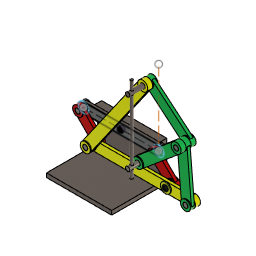
mechanism (Autodesk Fusion 360 design; units mm, degrees)
Autodesk Fusion 360 part; units mm, degrees
sketch "holder" plane through (0, 0, 0) normal (0, 1, 0) x (1, 0, 0) in component "holder"
  line L0 (-37.5, -5) -> (37.5, -5)
  arc A0 (37.5, -5) -> (37.5, 5) centre (37.5, 0) ccw
  line L1 (37.5, 5) -> (-37.5, 5)
  arc A1 (-37.5, 5) -> (-37.5, -5) centre (-37.5, 0) ccw
  line L2 (-37.5, 0) -> (37.5, 0) construction
  circle A2 centre (-37.5, 0) radius 5
  circle A3 centre (-37.5, 0) radius 2.5
  circle A4 centre (37.5, 0) radius 5
  circle A5 centre (37.5, 0) radius 2.5
  line L3 (37.5, 0) -> (37.5, -75) construction
  dimension "d1" = 10
  dimension "d2" = 10
  dimension "d3" = 5
  constraint tangent L0 A0
  constraint tangent A0 L1
  constraint parallel L0 L1
  constraint tangent L1 A1
  constraint tangent L0 A1
  constraint horizontal L2
  constraint midpoint L2 origin
  constraint concentric A1 A2
  constraint concentric A2 A3
  constraint concentric A0 A4
  constraint concentric A4 A5
  constraint coincident A0.centre L2.end
  constraint perpendicular L2 L3
  measures "d1" diameter of A0
  measures "d2" diameter of A2
  measures "d3" diameter of A3
extrude "Extrude1" add sketch "holder" along normal blind 3 makes body 1 in component "holder"
extrude "Extrude2" add sketch "holder" along normal blind 4 and the other way blind 1 contours A1 A2 | A0 A4 bodies 1 in component "holder"
sketch "piece" plane through (0, -1, 0) normal (0, -1, 0) x (1, 0, 0) in component "left red"
  circle A0 centre (-37.5, 0) radius 2.5
  circle A1 centre (-37.5, 0) radius 5
  line L0 (-41.0355, -3.5355) -> (-23.3579, -21.2132)
  arc A2 (-23.3579, -21.2132) -> (-16.2868, -14.1421) centre (-19.8223, -17.6777) ccw
  line L1 (-16.2868, -14.1421) -> (-33.9645, 3.5355)
  arc A3 (-33.9645, 3.5355) -> (-41.0355, -3.5355) centre (-37.5, 0) ccw
  line L2 (-37.5, 0) -> (-19.8223, -17.6777) construction
  circle A4 centre (-37.5, 0) radius 5
  circle A5 centre (-37.5, 0) radius 2.5
  circle A6 centre (-19.8223, -17.6777) radius 5
  circle A7 centre (-19.8223, -17.6777) radius 2.5
  dimension "d10" = 10
  dimension "d11" = 5
  constraint tangent L0 A2
  constraint tangent A2 L1
  constraint parallel L0 L1
  constraint tangent L1 A3
  constraint tangent L0 A3
  constraint coincident A0.centre A1.centre
  constraint concentric A3 A4
  constraint concentric A4 A5
  constraint concentric A2 A6
  constraint concentric A2 A7
  measures "d10" diameter of A2
  measures "d11" diameter of A7
extrude "Extrude1'" add sketch "piece" along normal blind 4 and the other way blind -1 separate body makes body 2 in component "left red"
extrude "Extrude2'" add sketch "piece" along normal blind 5 contours A1 A3 A4 | A2 A6 bodies 2 in component "left red"
sketch "piece (2)" plane through (0, -1, 0) normal (0, -1, 0) x (1, 0, 0) in component "right red"
  circle A0 centre (-37.5, 0) radius 2.5
  circle A1 centre (-37.5, 0) radius 5
  line L0 (-41.0355, -3.5355) -> (-23.3579, -21.2132)
  arc A2 (-23.3579, -21.2132) -> (-16.2868, -14.1421) centre (-19.8223, -17.6777) ccw
  line L1 (-16.2868, -14.1421) -> (-33.9645, 3.5355)
  arc A3 (-33.9645, 3.5355) -> (-41.0355, -3.5355) centre (-37.5, 0) ccw
  line L2 (-37.5, 0) -> (-19.8223, -17.6777) construction
  circle A4 centre (-37.5, 0) radius 5
  circle A5 centre (-37.5, 0) radius 2.5
  circle A6 centre (-19.8223, -17.6777) radius 5
  circle A7 centre (-19.8223, -17.6777) radius 2.5
  dimension "d10_1" = 10
  dimension "d11_1" = 5
  constraint tangent L0 A2
  constraint tangent A2 L1
  constraint parallel L0 L1
  constraint tangent L1 A3
  constraint tangent L0 A3
  constraint coincident A0.centre A1.centre
  constraint concentric A3 A4
  constraint concentric A4 A5
  constraint concentric A2 A6
  constraint concentric A2 A7
  measures "d10_1" diameter of A2
  measures "d11_1" diameter of A7
extrude "Extrude1''" add sketch "piece (2)" along normal blind 4 and the other way blind -1 separate body makes body 3 in component "right red"
extrude "Extrude2''" add sketch "piece (2)" along normal blind 5 contours A1 A3 A4 | A2 A6 bodies 3 in component "right red"
sketch "piece (3)" plane through (0, -6, 0) normal (0, -1, 0) x (1, 0, 0) in component "bottom yellow"
  circle A0 centre (-19.8223, -17.6777) radius 2.5
  circle A1 centre (-19.8223, -17.6777) radius 5
  line L0 (-19.8223, -22.6777) -> (80.1777, -22.6777)
  arc A2 (80.1777, -22.6777) -> (80.1777, -12.6777) centre (80.1777, -17.6777) ccw
  line L1 (80.1777, -12.6777) -> (-19.8223, -12.6777)
  arc A3 (-19.8223, -12.6777) -> (-19.8223, -22.6777) centre (-19.8223, -17.6777) ccw
  line L2 (-19.8223, -17.6777) -> (80.1777, -17.6777) construction
  circle A4 centre (-19.8223, -17.6777) radius 5
  circle A5 centre (-19.8223, -17.6777) radius 2.5
  circle A6 centre (80.1777, -17.6777) radius 5
  circle A7 centre (80.1777, -17.6777) radius 2.5
  line L3 (80.1777, -17.6777) -> (55.1777, -17.6777) construction
  circle A8 centre (55.1777, -17.6777) radius 5
  circle A9 centre (55.1777, -17.6777) radius 2.5
  dimension "d18" = 100
  dimension "d19" = 10
  dimension "d20" = 5
  dimension "d21" = 25
  dimension "d22" = 10
  dimension "d23" = 5
  constraint tangent L0 A2
  constraint tangent A2 L1
  constraint parallel L0 L1
  constraint tangent L1 A3
  constraint tangent L0 A3
  constraint horizontal L2
  constraint coincident A0.centre A1.centre
  constraint concentric A3 A4
  constraint concentric A3 A5
  constraint concentric A2 A6
  constraint concentric A6 A7
  constraint coincident A2.centre L2.end
  constraint coincident L2 L3.end
  constraint coincident L3.end A8.centre
  constraint concentric A8 A9
  measures "d18" distance of A0.centre A2.centre
  measures "d19" diameter of A2
  measures "d20" diameter of A7
  measures "d21" distance of A2.centre L3.end
  measures "d22" diameter of A8
  measures "d23" diameter of A9
extrude "Extrude1'''" add sketch "piece (3)" along normal blind 4 and the other way blind -1 separate body makes body 4 in component "bottom yellow"
extrude "Extrude2'''" add sketch "piece (3)" along normal blind 5 contours A1 A3 A4 | A8 | A2 A6 bodies 4 in component "bottom yellow"
sketch "piece (4)" plane through (0, -11, 0) normal (0, -1, 0) x (1, 0, 0) in component "top yellow"
  circle A0 centre (-19.8223, -17.6777) radius 2.5
  circle A1 centre (-19.8223, -17.6777) radius 5
  line L0 (-15.7253, -20.5438) -> (41.597, 61.3961)
  arc A2 (41.597, 61.3961) -> (33.403, 67.1284) centre (37.5, 64.2623) ccw
  line L1 (33.403, 67.1284) -> (-23.9193, -14.8116)
  arc A3 (-23.9193, -14.8116) -> (-15.7253, -20.5438) centre (-19.8223, -17.6777) ccw
  line L2 (-19.8223, -17.6777) -> (37.5, 64.2623) construction
  line L3 (37.5, 0) -> (37.5, 75)
  circle A4 centre (-19.8223, -17.6777) radius 5
  circle A5 centre (-19.8223, -17.6777) radius 2.5
  circle A6 centre (37.5, 64.2623) radius 5
  circle A7 centre (37.5, 64.2623) radius 2.5
  dimension "d30" = 100
  dimension "d31" = 10
  dimension "d32" = 5
  constraint tangent L0 A2
  constraint tangent A2 L1
  constraint parallel L0 L1
  constraint tangent L1 A3
  constraint tangent L0 A3
  constraint coincident A0.centre A1.centre
  constraint coincident A2.centre L3
  constraint concentric A3 A4
  constraint concentric A3 A5
  constraint concentric A2 A6
  constraint concentric A2 A7
  measures "d30" distance of A0.centre A2.centre
  measures "d31" diameter of A2
  measures "d32" diameter of A7
extrude "Extrude1''''" add sketch "piece (4)" along normal blind 4 and the other way blind -1 separate body contours A1 A3 A4 | A1 L0 L1 L3 A4 A6 | A2 L3 A6 A7 | L0 L3 A6 | A2 L3 A6 A7 makes body 5 in component "top yellow"
extrude "Extrude2''''" add sketch "piece (4)" along normal blind 5 contours A1 A3 A4 | A2 L3 A6 A7 | A2 L3 A6 A7 bodies 5 in component "top yellow"
sketch "piece (5)" plane through (0, -11, 0) normal (0, -1, 0) x (1, 0, 0) in component "right green"
  circle A0 centre (80.1777, -17.6777) radius 2.5
  circle A1 centre (80.1777, -17.6777) radius 5
  line L0 (85.1586, -17.2419) -> (80.8009, 32.5678)
  arc A2 (80.8009, 32.5678) -> (70.8389, 31.6963) centre (75.8199, 32.1321) ccw
  line L1 (70.8389, 31.6963) -> (75.1967, -18.1134)
  arc A3 (75.1967, -18.1134) -> (85.1586, -17.2419) centre (80.1777, -17.6777) ccw
  line L2 (80.1777, -17.6777) -> (75.8199, 32.1321) construction
  line L3 (80.1777, -17.6777) -> (130.1777, -17.6777) construction
  circle A4 centre (80.1777, -17.6777) radius 5
  circle A5 centre (80.1777, -17.6777) radius 2.5
  circle A6 centre (75.8199, 32.1321) radius 5
  circle A7 centre (75.8199, 32.1321) radius 2.5
  dimension "d39" = 50
  dimension "d40" = 95
  dimension "d41" = 10
  dimension "d42" = 5
  constraint tangent L0 A2
  constraint tangent A2 L1
  constraint parallel L0 L1
  constraint tangent L1 A3
  constraint tangent L0 A3
  constraint coincident A0.centre A1.centre
  constraint concentric A3 A4
  constraint coincident L0.start A4
  constraint concentric A4 A5
  constraint concentric A2 A6
  constraint coincident L0.end A6
  constraint concentric A6 A7
  measures "d39" distance of A0.centre A2.centre
  measures "d40" angle of L2 L3
  measures "d41" diameter of A2
  measures "d42" diameter of A7
extrude "Extrude1'''''" add sketch "piece (5)" along normal blind 4 and the other way blind -1 separate body makes body 6 in component "right green"
extrude "Extrude2'''''" add sketch "piece (5)" along normal blind 5 contours A1 A3 A4 | A2 A6 bodies 6 in component "right green"
sketch "piece (6)" plane through (0, -11, 0) normal (0, 1, 0) x (-1, 0, 0) in component "top green"
  circle A0 centre (-37.5, 64.2623) radius 2.5
  circle A1 centre (-37.5, 64.2623) radius 5
  line L0 (-40.7125, 68.0937) -> (-79.0324, 35.9635)
  arc A2 (-79.0324, 35.9635) -> (-72.6074, 28.3007) centre (-75.8199, 32.1321) ccw
  line L1 (-72.6074, 28.3007) -> (-34.2875, 60.4308)
  arc A3 (-34.2875, 60.4308) -> (-40.7125, 68.0937) centre (-37.5, 64.2623) ccw
  line L2 (-37.5, 64.2623) -> (-75.8199, 32.1321) construction
  circle A4 centre (-75.8199, 32.1321) radius 5
  circle A5 centre (-75.8199, 32.1321) radius 2.5
  circle A6 centre (-37.5, 64.2623) radius 5
  circle A7 centre (-37.5, 64.2623) radius 2.5
  point P0 (-75.8199, 32.1321)
  dimension "d49" = 10
  dimension "d50" = 10
  dimension "d51" = 5
  constraint tangent L0 A2
  constraint tangent A2 L1
  constraint parallel L0 L1
  constraint tangent L1 A3
  constraint tangent L0 A3
  constraint coincident A0.centre A1.centre
  constraint coincident P0 A2.centre
  constraint concentric A4 A5
  constraint concentric A0 A6
  constraint concentric A6 A7
  measures "d49" diameter of A2
  measures "d50" diameter of A4
  measures "d51" diameter of A5
extrude "Extrude1''''''" add sketch "piece (6)" along normal blind 4 and the other way blind -1 separate body makes body 7 in component "top green"
extrude "Extrude2''''''" add sketch "piece (6)" along normal blind 5 contours A1 A3 A6 | A2 A4 bodies 7 in component "top green"
sketch "piece (7)" plane through (0, -16, 0) normal (0, -1, 0) x (1, 0, 0) in component "middle green"
  circle A0 centre (75.8199, 32.1321) radius 2.5
  circle A1 centre (75.8199, 32.1321) radius 5
  line L0 (72.6072, 35.9634) -> (34.2874, 3.8313)
  arc A2 (34.2874, 3.8313) -> (40.7126, -3.8313) centre (37.5, 0) ccw
  line L1 (40.7126, -3.8313) -> (79.0325, 28.3008)
  arc A3 (79.0325, 28.3008) -> (72.6072, 35.9634) centre (75.8199, 32.1321) ccw
  line L2 (75.8199, 32.1321) -> (37.5, 0) construction
  circle A4 centre (37.5, 0) radius 5
  circle A5 centre (37.5, 0) radius 2.5
  circle A6 centre (75.8199, 32.1321) radius 5
  circle A7 centre (75.8199, 32.1321) radius 2.5
  point P0 (37.5, 0)
  dimension "d58" = 10
  dimension "d59" = 10
  dimension "d60" = 5
  dimension "d61" = 10
  constraint tangent L0 A2
  constraint tangent A2 L1
  constraint parallel L0 L1
  constraint tangent L1 A3
  constraint tangent L0 A3
  constraint coincident A0.centre A1.centre
  constraint coincident P0 A2.centre
  constraint concentric A2 A4
  constraint concentric A3 A6
  constraint concentric A6 A7
  measures "d58" diameter of A2
  measures "d59" diameter of A4
  measures "d60" diameter of A5
  measures "d61" diameter of A6
extrude "Extrude1'''''''" add sketch "piece (7)" along normal blind 4 and the other way blind -1 separate body makes body 8 in component "middle green"
extrude "Extrude2'''''''" add sketch "piece (7)" along normal blind 5 contours A1 A3 A6 | A2 A4 bodies 8 in component "middle green"
sketch "holder (2)" plane through (0, -1, 0) normal (0, -1, 0) x (1, 0, 0) in component "link right red + middle green"
  circle A0 centre (37.5, 0) radius 2.5
  circle A1 centre (37.5, 0) radius 5
  circle A2 centre (37.5, 0) radius 2.2
  dimension "d68" = -0.3
extrude "Extrude1''''''''" add sketch "holder (2)" along normal blind 30 separate body contours A2 makes body 9 in component "link right red + middle green"
sketch "hole" plane through (0, 0, 0) normal (0, 0, 1) x (1, 0, 0) in component "link right red + middle green"
  line L0 (35, -27) -> (40, -27) construction
  circle A0 centre (37.5, -27) radius 1.5
  dimension "d71" = 3
  constraint horizontal L0
  constraint midpoint L0 A0.centre
  measures "d71" diameter of A0
sketch "holder (3)" plane through (0, -16, 0) normal (0, -1, 0) x (1, 0, 0) in component "link yellow + top green"
  circle A0 centre (37.5, 64.2623) radius 2.5
  circle A1 centre (37.5, 64.2623) radius 5
  circle A2 centre (37.5, 64.2623) radius 2.2
  dimension "d72" = -0.3
extrude "Extrude1'''''''''" add sketch "holder (3)" along normal blind -10 and the other way blind -15 separate body contours A2 makes body 10 in component "link yellow + top green"
sketch "stick" plane through (0, 0, 0) normal (0, 0, 1) x (1, 0, 0) in component "link yellow + top green"
  circle A0 centre (37.5, -27) radius 1.35
  point P0 (37.5, -27)
  dimension "d138" = 2.7
  constraint coincident P0 A0.centre
  measures "d138" diameter of A0
extrude "Extrude3" add sketch "stick" along normal blind 75 and the other way blind 10 bodies 10 in component "link yellow + top green"
extrude "Extrude3'" cut sketch "hole" along normal blind 9 and the other way blind 4 bodies 9 in component "link right red + middle green"
sketch "link" plane through (0, -6, 0) normal (0, -1, 0) x (1, 0, 0) in component "link - holder + left red"
  circle A0 centre (-37.5, 0) radius 2.5
  circle A1 centre (-37.5, 0) radius 5
  circle A2 centre (-37.5, 0) radius 2.35
  dimension "d171" = 4.7
  constraint concentric A0 A2
  measures "d171" diameter of A2
extrude "Extrude1''''''''''" add sketch "link" against normal blind 10 separate body contours A2 makes body 11 in component "link - holder + left red"
sketch "link (2)" plane through (0, -6, 0) normal (0, -1, 0) x (1, 0, 0) in component "link - right red + bottom yellow"
  circle A0 centre (-37.5, 0) radius 2.5
  circle A1 centre (-37.5, 0) radius 5
  circle A2 centre (-37.5, 0) radius 2.35
  dimension "d171_1" = 4.7
  constraint concentric A0 A2
  measures "d171_1" diameter of A2
extrude "Extrude1'''''''''''" add sketch "link (2)" against normal blind 10 separate body contours A2 makes body 12 in component "link - right red + bottom yellow"
sketch "link (3)" plane through (0, -6, 0) normal (0, -1, 0) x (1, 0, 0) in component "link - bottom yellow + right green"
  circle A0 centre (-37.5, 0) radius 2.5
  circle A1 centre (-37.5, 0) radius 5
  circle A2 centre (-37.5, 0) radius 2.35
  dimension "d171_1_1" = 4.7
  constraint concentric A0 A2
  measures "d171_1_1" diameter of A2
extrude "Extrude1''''''''''''" add sketch "link (3)" against normal blind 10 separate body contours A2 makes body 13 in component "link - bottom yellow + right green"
sketch "link (4)" plane through (0, -16, 0) normal (0, -1, 0) x (1, 0, 0) in component "link - yellows + left red"
  circle A0 centre (-19.8223, -17.6777) radius 2.5
  circle A1 centre (-19.8223, -17.6777) radius 5
  circle A2 centre (-19.8223, -17.6777) radius 2.35
  dimension "d174" = 4.7
  constraint concentric A0 A2
  measures "d174" diameter of A2
extrude "Extrude1'''''''''''''" add sketch "link (4)" against normal blind 15 separate body contours A2 makes body 14 in component "link - yellows + left red"
sketch "link (5)" plane through (0, -16, 0) normal (0, -1, 0) x (1, 0, 0) in component "link - greens"
  circle A0 centre (-19.8223, -17.6777) radius 2.5
  circle A1 centre (-19.8223, -17.6777) radius 5
  circle A2 centre (-19.8223, -17.6777) radius 2.35
  dimension "d174_1" = 4.7
  constraint concentric A0 A2
  measures "d174_1" diameter of A2
extrude "Extrude1''''''''''''''" add sketch "link (5)" against normal blind 15 separate body contours A2 makes body 15 in component "link - greens"
extrude "Extrude4" add sketch "holder (2)" against normal blind 5 contours A2 bodies 9 in component "link right red + middle green"
sketch "floor holder" plane through (0, 3, 0) normal (0, 1, 0) x (-1, 0, 0) in component "holder"
  arc A0 (-37.5, -5) -> (-37.5, 5) centre (-37.5, 0) ccw
  line L0 (-37.5, -5) -> (37.5, -5)
  arc A1 (37.5, 5) -> (37.5, -5) centre (37.5, 0) ccw
  line L1 (37.5, 5) -> (-37.5, 5)
  line L2 (32.5, 5) -> (-32.5, 5)
  line L3 (-32.5, 5) -> (-32.5, -5)
  line L4 (-32.5, -5) -> (32.5, -5)
  line L5 (32.5, -5) -> (32.5, 5)
  line L6 (32.5, 5) -> (-32.5, -5) construction
  line L7 (-32.5, 5) -> (32.5, -5) construction
  dimension "d179" = 65
  constraint horizontal L2
  constraint perpendicular L2 L3
  constraint parallel L2 L4
  constraint parallel L3 L5
  constraint coincident L6 origin
  constraint coincident L7 origin
  measures "d179" distance of L3.end L4.end
extrude "Extrude3''" add sketch "floor holder" along normal blind 20 separate body contours L0 L1 L2 L3 L4 L5 makes body 16 in component "holder"
extrude "Extrude4'" cut 1 faces at (-10.8333, 16.3333, 5) along direction (0, 0, -1) blind 3 on bodies 16 bodies 16 in component "holder"
extrude "Extrude5" cut 1 faces at (10.8333, 16.3333, -5) along direction (0, 0, 1) blind 3 on bodies 16 bodies 16 in component "holder"
sketch "vertical" plane through (0, 0, -2) normal (0, 0, -1) x (1, 0, 0) in component "holder"
  line L0 (32.5, -3) -> (-32.5, -3)
  line L1 (-32.5, -3) -> (-32.5, -23)
  line L2 (-32.5, -23) -> (32.5, -23)
  line L3 (32.5, -23) -> (32.5, -3)
  line L4 (-32.5, -13) -> (32.5, -13)
  line L5 (32.5, -13) -> (32.5, -9)
  line L6 (32.5, -9) -> (-32.5, -9)
  line L7 (-32.5, -9) -> (-32.5, -13)
  line L8 (-32.5, -13) -> (32.5, -9) construction
  line L9 (32.5, -13) -> (-32.5, -9) construction
  point P0 (0, -11)
  constraint horizontal L4
  constraint perpendicular L4 L5
  constraint parallel L4 L6
  constraint parallel L5 L7
  constraint midpoint L1 L4.start
  constraint coincident L8 P0
  constraint coincident L9 P0
extrude "Extrude6" add sketch "vertical" along normal blind 35 contours L1 L3 L4 L5 L6 L7 bodies 16 in component "holder"
sketch "horizontal" plane through (0, 13, 0) normal (0, 1, 0) x (-1, 0, 0) in component "holder"
  line L0 (32.5, -2) -> (-32.5, -2)
  line L1 (-32.5, -2) -> (-32.5, -37)
  line L2 (-32.5, -37) -> (32.5, -37)
  line L3 (32.5, -37) -> (32.5, -2)
  line L4 (-32.5, -37) -> (32.5, -37)
  line L5 (32.5, -37) -> (32.5, -33)
  line L6 (32.5, -33) -> (-32.5, -33)
  line L7 (-32.5, -33) -> (-32.5, -37)
  dimension "d188" = 4
  constraint horizontal L4
  constraint vertical L5
  constraint horizontal L6
  constraint vertical L7
  constraint coincident L1.end L2.start
  measures "d188" distance of L1.end L6.end
extrude "Extrude7" add sketch "horizontal" along normal blind -55 and the other way blind -10 contours L1 L2 L3 L4 L5 L6 L7 bodies 16 in component "holder"
extrude "Extrude8" cut 2 faces at (10.8333, 23, -35.6667) (10.8333, 23, 0.6667) along direction (0, -1, 0) blind 10 on bodies 16 bodies 16 in component "holder"
combine "Combine1" operation add target body 16 tool bodies 1 in component "holder"
component "holder" placed x (1, 0, 0) y (0, 1, 0) z (0, 0, 1) at (0, 0, 0)
component "left red" placed x (1, 0, 0) y (0, 1, 0) z (0, 0, 1) at (0, 0, 0)
component "right red" placed x (1, 0, 0) y (0, 1, 0) z (0, 0, 1) at (75, 0, 0)
component "bottom yellow" placed x (1, 0, 0) y (0, 1, 0) z (0, 0, 1) at (0, 0, 0)
component "top yellow" placed x (1, 0, 0) y (0, 1, 0) z (0, 0, 1) at (0, 0, 0)
component "right green" placed x (1, 0, 0) y (0, 1, 0) z (0, 0, 1) at (0, 0, 0)
component "top green" placed x (1, 0, 0) y (0, 1, 0) z (0, 0, 1) at (0, 0, 0)
component "middle green" placed x (1, 0, 0) y (0, 1, 0) z (0, 0, 1) at (0, 0, 0)
component "links" placed x (1, 0, 0) y (0, 1, 0) z (0, 0, 1) at (0, 0, 0)
component "link - greens" placed x (1, 0, 0) y (0, 1, 0) z (0, 0, 1) at (95.6422, -5, 49.8097) in component "links"
component "link - yellows + left red" placed x (1, 0, 0) y (0, 1, 0) z (0, 0, 1) at (0, 0, 0) in component "links"
component "link - bottom yellow + right green" placed x (1, 0, 0) y (0, 1, 0) z (0, 0, 1) at (117.6777, -10, -17.6777) in component "links"
component "link - right red + bottom yellow" placed x (1, 0, 0) y (0, 1, 0) z (0, 0, 1) at (92.6777, -5, -17.6777) in component "links"
component "link - holder + left red" placed x (1, 0, 0) y (0, 1, 0) z (0, 0, 1) at (0, 0, 0) in component "links"
component "link yellow + top green" placed x (1, 0, 0) y (0, 1, 0) z (0, 0, 1) at (0, 0, 0) in component "links"
component "link right red + middle green" placed x (1, 0, 0) y (0, 1, 0) z (0, 0, 1) at (0, 0, 0) in component "links"
equation "d138 = 3 mm - 0.3 mm"
equation "d171 = 5 mm - 0.3 mm"
equation "d171_1 = 5 mm - 0.3 mm"
equation "d171_1_1 = 5 mm - 0.3 mm"
equation "d174 = 5 mm - 0.3 mm"
equation "d174_1 = 5 mm - 0.3 mm"
named bodies: "holder", "piece", "link"
